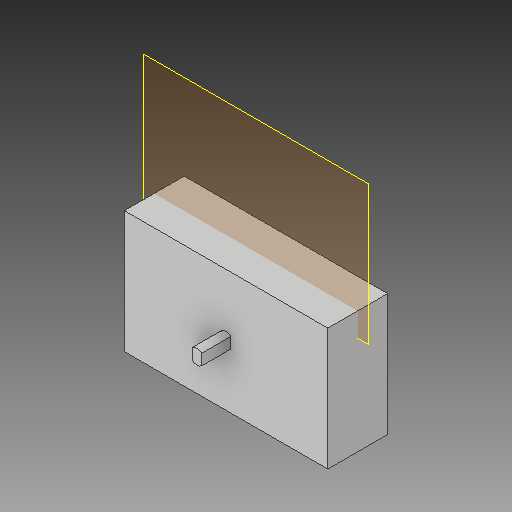
# Autodesk Inventor part: Geared_Motor
Saved by Autodesk Inventor 2019 (Build 230136000, 136)
## iProperties
Created: 2019-02-26
Part Number: Geared_Motor
Material: Generic
Document SubType Name: Modeling
Designer: alarr
Density: 1 g/cm^3
Appearance: Default
Author: alarr
Autodesk Inventor part; units mm, degrees
ref_plane "YZ Plane" through (0, 0, 0) normal (1, 0, 0) x (0, 1, 0)
ref_plane "XZ Plane" through (0, 0, 0) normal (0, 1, 0) x (-1, 0, 0)
ref_plane "XY Plane" through (0, 0, 0) normal (0, 0, 1) x (1, 0, 0)
sketch "Sketch1" plane through (0, 0, 0) normal (0, 0, 1) x (1, 0, 0)
  arc A0 (1.778, -29.9361) -> (-1.778, -29.9361) centre (0, -31.75) ccw construction
  line L0 (1.778, -29.9361) -> (1.778, -33.5639) construction
  arc A1 (-1.778, -33.5639) -> (1.778, -33.5639) centre (0, -31.75) ccw construction
  line L1 (-1.778, -33.5639) -> (-1.778, -29.9361) construction
  line L2 (1.778, -29.9361) -> (1.778, -33.5639) construction
  line L3 (-1.778, -29.9361) -> (-1.778, -33.5639) construction
  arc A2 (1.778, -29.9361) -> (-1.778, -29.9361) centre (0, -31.75) ccw construction
  arc A3 (-1.778, -33.5639) -> (1.778, -33.5639) centre (0, -31.75) ccw construction
  arc A4 (1.524, -30.0461) -> (-1.524, -30.0461) centre (0, -31.75) ccw
  line L4 (1.524, -30.0461) -> (1.524, -33.4539)
  arc A5 (-1.524, -33.4539) -> (1.524, -33.4539) centre (0, -31.75) ccw
  line L5 (-1.524, -33.4539) -> (-1.524, -30.0461)
  point P0 (0, 0)
  point P1 (0, -34.29)
  point P2 (0, -29.21)
  dimension "d0" = 0.254
  constraints: 12 point on circle, 8 end point, 4 centre point, 1 parallel, 1 vertical, 3 other
  measures "d0" radial gap between concentric circles of A0 A4
extrude "Extrusion1" add sketch "Sketch1" along normal mid plane 36.83
ref_plane "Work Plane1" through (0, 0, 0) normal (0, 0, 1) x (1, 0, 0)
sketch "Sketch2" plane through (0, 0, 0) normal (0, 0, 1) x (1, 0, 0)
  line L0 (31.75, -50.8) -> (-31.75, -50.8)
  line L1 (-31.75, -50.8) -> (-31.75, -12.7)
  line L2 (-31.75, -12.7) -> (31.75, -12.7)
  line L3 (31.75, -12.7) -> (31.75, -50.8)
  line L4 (31.75, -50.8) -> (-31.75, -12.7) construction
  line L5 (-31.75, -50.8) -> (31.75, -12.7) construction
  circle A0 centre (0, -31.75) radius 5.715 projected
  dimension "d5" = 63.5
  dimension "d6" = 38.1
  constraints: 12 end point, 2 midpoint, 2 parallel, 1 coincident, 1 horizontal, 1 perpendicular
  measures "d5" distance of L1.end L2.end
  measures "d6" distance of L0.end L1.end
extrude "Extrusion2" add sketch "Sketch2" along normal mid plane 18.669 contours L0 L1 L2 L3 | A0
body "Solid1"
